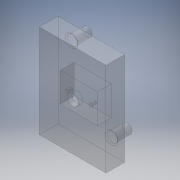
# Autodesk Inventor part: Base-Cover
Saved by Autodesk Inventor 2019 (Build 230136000, 136)
## iProperties
Created: 2021-01-07
Part Number: Base-Cover
Material: Polycarbonate, Clear
Document SubType Name: Modeling
Designer: Sam
Density: 1.2 g/cm^3
Appearance: Polycarbonate - Clear
Author: Sam
Autodesk Inventor part; units mm, degrees
ref_plane "YZ Plane" through (0, 0, 0) normal (1, 0, 0) x (0, 1, 0)
ref_plane "XZ Plane" through (0, 0, 0) normal (0, 1, 0) x (-1, 0, 0)
ref_plane "XY Plane" through (0, 0, 0) normal (0, 0, 1) x (1, 0, 0)
sketch "Sketch1" plane through (0, 0, 0) normal (0, 0, 1) x (1, 0, 0)
  line L0 (-12.5, -17.5) -> (12.5, -17.5) projected
  line L1 (12.5, -17.5) -> (12.5, 17.5) projected
  line L2 (-12.5, 17.5) -> (-12.5, -17.5) projected
  line L3 (12.5, 17.5) -> (-12.5, 17.5) projected
  circle A0 centre (0, 0) radius 2.05
  dimension "d0" = 4.1
  constraints: 1 centre point, 1 coincident
  measures "d0" diameter of A0
extrude "Extrusion1" add sketch "Sketch1" along normal blind 7
sketch "Sketch2" plane through (0, 0, 0) normal (0, 0, -1) x (-1, 0, 0)
  circle A0 centre (-8, -12) radius 2.1 projected
  circle A1 centre (7, 12) radius 2.1 projected
  circle A2 centre (-8, -12) radius 1.9
  circle A3 centre (7, 12) radius 1.9
  dimension "d9" = 3.8
  constraints: 2 centre point, 2 coincident, 1 equal radius
  measures "d9" diameter of A2
extrude "Extrusion3" add sketch "Sketch2" along normal blind 6 draft -1 contours A2 | A3
sketch "Sketch3" plane through (0, 0, 0) normal (0, 0, -1) x (-1, 0, 0)
  line L0 (5.5902, -5) -> (-5.5902, -5) construction
  line L1 (-5.5902, 5) -> (5.5902, 5) construction
  line L2 (-7, -5.2) -> (7, -5.2)
  line L3 (7, -5.2) -> (7, 5.2)
  line L4 (7, 5.2) -> (-7, 5.2)
  line L5 (-7, 5.2) -> (-7, -5.2)
  line L6 (-6, -4.5) -> (-6, 4.5) construction
  line L7 (6, 4.5) -> (6, -4.5) construction
  line L8 (-5.5902, 5) -> (5.5902, 5) projected
  line L9 (5.5902, -5) -> (-5.5902, -5) projected
  dimension "d28" = 1
  dimension "d29" = 1
  dimension "d30" = 0.2
  dimension "d31" = 0.2
  constraints: 8 end point, 2 parallel, 1 horizontal, 1 perpendicular
  measures "d28" distance between parallel lines of L6 L5
  measures "d29" distance between parallel lines of L3 L7
  measures "d30" distance between parallel lines of L1 L4
  measures "d31" distance between parallel lines of L2 L0
extrude "Extrusion4" cut sketch "Sketch3" against normal blind 5.2
sketch "Sketch4" plane through (0, 0, 5.2) normal (0, 0, -1) x (-1, 0, 0)
  circle A0 centre (-4.5, 0) radius 0.6105 projected
  circle A1 centre (4.5, 0) radius 0.6105 projected
  circle A2 centre (-4.5, 0) radius 0.5
  circle A3 centre (4.5, 0) radius 0.5
  point P0 (0, 0)
  dimension "d18" = 1
  constraints: 4 coincident, 2 centre point, 1 equal radius
  measures "d18" diameter of A2
extrude "Extrusion5" add sketch "Sketch4" along normal blind 2 contours A2 | A3
fillet "Fillet1" radius 0.2 2 edges at (-4, 0, 5.2) (5, 0, 5.2)
fillet "Fillet2" radius 0.4 2 edges at (-4, 0, 3.2) (5, 0, 3.2)
fillet "Fillet3" radius 0.5 2 edges at (-5.1, 12, 0) (9.9, -12, 0)
body "Solid1"
